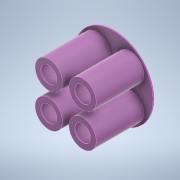
# Autodesk Inventor part: Cam Barrel Plate (printable)
Saved by Autodesk Inventor 2022.2 (Build 262287030, 287C)
## iProperties
Created: 2022-02-09
Part Number: Cam Barrel Plate (printable)
Material: ABS Plastic
Document SubType Name: Modeling
Designer: smiku
Density: 1.06 g/cm^3
Appearance: Smooth - Purple
Author: smiku
Autodesk Inventor part; units mm, degrees
ref_plane "YZ Plane" through (0, 0, 0) normal (1, 0, 0) x (0, 1, 0)
ref_plane "XZ Plane" through (0, 0, 0) normal (0, 1, 0) x (-1, 0, 0)
ref_plane "XY Plane" through (0, 0, 0) normal (0, 0, 1) x (1, 0, 0)
sketch "Sketch1" plane through (0, 0, 0) normal (0, 0, 1) x (1, 0, 0)
  circle A0 centre (0, 0) radius 50
  circle A1 centre (21.2132, 21.2132) radius 16
  circle A2 centre (21.2132, 21.2132) radius 17.2
  line L0 (0, 0) -> (50, 0) construction
  line L1 (0, 0) -> (35.3553, 35.3553) construction
  circle A3 centre (-21.2132, 21.2132) radius 16
  circle A4 centre (-21.2132, 21.2132) radius 17.2
  circle A5 centre (-21.2132, -21.2132) radius 16
  circle A6 centre (-21.2132, -21.2132) radius 17.2
  circle A7 centre (21.2132, -21.2132) radius 16
  circle A8 centre (21.2132, -21.2132) radius 17.2
  dimension "d0" = 32
  dimension "d2" = 100
  dimension "d3" = 1.2
  dimension "d5" = 45
  dimension "d6" = 30
  dimension "d9" = 360
  constraints: 9 centre point, 4 end point, 2 coincident, 2 point on circle, 1 horizontal, 1 point on line, 13 other
  measures "d0" diameter of A1
  measures "d2" diameter of A0
  measures "d3" radial gap between concentric circles of A2 A1
  measures "d5" angle of L0 L1
  measures "d6" distance of L0.start A1.centre
extrude "Extrusion1" add sketch "Sketch1" against normal blind 1.2 contours A0 | A2 | A4 | A6 | A8
extrude "Extrusion2" add sketch "Sketch1" along normal blind 60 contours A2 | A4 | A6 | A8
sketch "Sketch2" plane through (21.2132, 21.2132, 60) normal (0, 0, 1) x (1, 0, 0)
  circle A0 centre (-42.4264, 0) radius 16 projected
  circle A1 centre (0, 0) radius 16 projected
  circle A2 centre (0, -42.4264) radius 16 projected
  circle A3 centre (-42.4264, -42.4264) radius 16 projected
  circle A4 centre (0, 0) radius 10.25
  circle A5 centre (-42.4264, 0) radius 10.25
  circle A6 centre (-42.4264, -42.4264) radius 10.25
  circle A7 centre (0, -42.4264) radius 10.25
  point P0 (-21.2132, -21.2132)
  dimension "d15" = 20.5
  constraints: 4 centre point, 3 equal radius, 1 coincident
  measures "d15" diameter of A4
extrude "Extrusion3" add sketch "Sketch2" against normal blind 1.2
body "Solid1"
